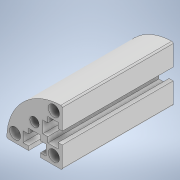
# Autodesk Inventor part: AFSR-2020-4-1000
Saved by Autodesk Inventor 2021.1 (Build 251245010, 245A)
## iProperties
Created: 2016-10-06
Part Number: AFSR-2020-4-1000
Material: 一般
Document SubType Name: Modeling
Designer: gisen
Density: 1 g/cm^3
Appearance: 既定
Sending System: Autodesk Inventor 2014
Preprocessor: ST-DEVELOPER v15.2
Title: C:\Users\AMS43\Documents\Inventor\AMS\misumi\フレーム_ipt\フレーム_stp\AFSR-2020-4.ipt.stp
Author: AMS43
Autodesk Inventor part; units mm, degrees
ref_plane "YZ Plane" through (0, 0, 0) normal (1, 0, 0) x (0, 1, 0)
ref_plane "XZ Plane" through (0, 0, 0) normal (0, 1, 0) x (-1, 0, 0)
ref_plane "作業平面1" through (2.15, -10, 1000) normal (0, 0, 1) x (1, 0, 0)
sketch "スケッチ1" plane through (2.15, -10, 1000) normal (0, 0, 1) x (1, 0, 0)
  line L0 (6.35, 12.15) -> (7.85, 12.15) projected
  line L1 (7.85, 12.15) -> (7.85, 19.4936) projected
  arc A0 (7.85, 19.4936) -> (7.3372, 19.9934) centre (7.35, 19.4936) ccw projected
  arc A1 (7.3372, 19.9934) -> (-12.1434, 0.5128) centre (7.85, 0) ccw projected
  arc A2 (-12.1434, 0.5128) -> (-11.6436, 0) centre (-11.6436, 0.5) ccw projected
  line L2 (-11.6436, 0) -> (-4.3, 0) projected
  line L3 (-4.3, 0) -> (-4.3, 1.5) projected
  line L4 (-4.3, 1.5) -> (-6.3, 1.5) projected
  line L5 (-6.3, 1.5) -> (-6.3, 5.2) projected
  line L6 (-6.3, 5.2) -> (-4.3, 5.2) projected
  line L7 (-4.3, 5.2) -> (-4.3, 7) projected
  line L8 (-4.3, 7) -> (0, 7) projected
  line L9 (0, 7) -> (0, 5.2) projected
  line L10 (0, 5.2) -> (2, 5.2) projected
  line L11 (2, 5.2) -> (2, 1.5) projected
  line L12 (2, 1.5) -> (0, 1.5) projected
  line L13 (0, 1.5) -> (0, 0) projected
  line L14 (0, 0) -> (7.35, 0) projected
  arc A3 (7.35, 0) -> (7.85, 0.5) centre (7.35, 0.5) ccw projected
  line L15 (7.85, 0.5) -> (7.85, 7.85) projected
  line L16 (7.85, 7.85) -> (6.35, 7.85) projected
  line L17 (6.35, 7.85) -> (6.35, 5.85) projected
  line L18 (6.35, 5.85) -> (2.65, 5.85) projected
  line L19 (2.65, 5.85) -> (2.65, 7.85) projected
  line L20 (2.65, 7.85) -> (0.85, 7.85) projected
  line L21 (0.85, 7.85) -> (0.85, 12.15) projected
  line L22 (0.85, 12.15) -> (2.65, 12.15) projected
  line L23 (2.65, 12.15) -> (2.65, 14.15) projected
  line L24 (2.65, 14.15) -> (6.35, 14.15) projected
  line L25 (6.35, 14.15) -> (6.35, 12.15) projected
  circle A4 centre (4.85, 3) radius 2 projected
  circle A5 centre (-9.15, 3) radius 2 projected
  circle A6 centre (4.85, 17) radius 2 projected
  circle A7 centre (-2.15, 10) radius 1.65 projected
extrude "押し出し1" add sketch "スケッチ1" along normal blind 40
